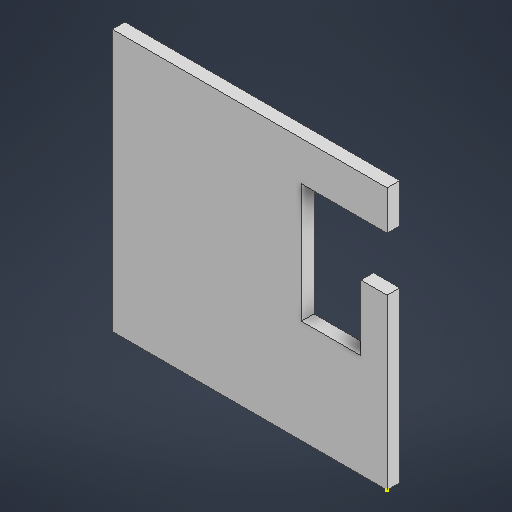
# Autodesk Inventor part: base1ek
Saved by Autodesk Inventor 2026.1 (Build 301233020, 233B)
## iProperties
Created: 2026-04-29
Part Number: base1ek
Material: Generic
Document SubType Name: Modeling
Designer: kadir
Density: 1 g/cm^3
Appearance: Default
Author: kadir
Autodesk Inventor part; units mm, degrees
ref_plane "YZ Plane" through (0, 0, 0) normal (1, 0, 0) x (0, 1, 0)
ref_plane "XZ Plane" through (0, 0, 0) normal (0, 1, 0) x (-1, 0, 0)
ref_plane "XY Plane" through (0, 0, 0) normal (0, 0, 1) x (1, 0, 0)
sketch "Sketch1" plane through (0, 0, 0) normal (0, 0, 1) x (1, 0, 0)
  line L0 (0, 0) -> (-210, 0)
  line L1 (-210, 0) -> (-210, 200)
  line L2 (-210, 200) -> (0, 200)
  line L3 (0, 200) -> (0, 0)
  line L4 (-65.5, 79) -> (-65.5, 170)
  line L5 (-65.5, 170) -> (0, 170)
  line L6 (-65.5, 79) -> (-20, 79)
  line L7 (-20, 79) -> (-20, 129)
  line L8 (-20, 129) -> (0, 129)
  line L9 (0, 129) -> (0, 170)
  point P0 (0, 149.5)
  point P1 (0, 129)
  dimension "d0" = 210
  dimension "d1" = 200
  dimension "d2" = 91
  dimension "d3" = 45.5
  dimension "d4" = 50
  dimension "d5" = 20
  dimension "d6" = 30
  constraints: 20 end point, 4 perpendicular, 2 horizontal, 2 parallel, 2 vertical, 1 midpoint, 1 vertical alignment
  measures "d0" distance of L1.end L2.end
  measures "d1" distance of L0.end L1.end
  measures "d2" distance of L4.start L4.end
  measures "d3" distance of L4.start L6.end
  measures "d4" distance of L6.end L7.end
  measures "d5" distance of L7.end L8.end
  measures "d6" distance between parallel lines of L5 L2
extrude "Extrusion1" add sketch "Sketch1" along normal blind 9.653 contours L0 L1 L2 L3 L5 L4 L6 L7 L8
sketch "Sketch2" plane through (0, 0, 9.653) normal (0, 0, 1) x (1, 0, 0)
  point P0 (0, 0)
body "Solid1"
